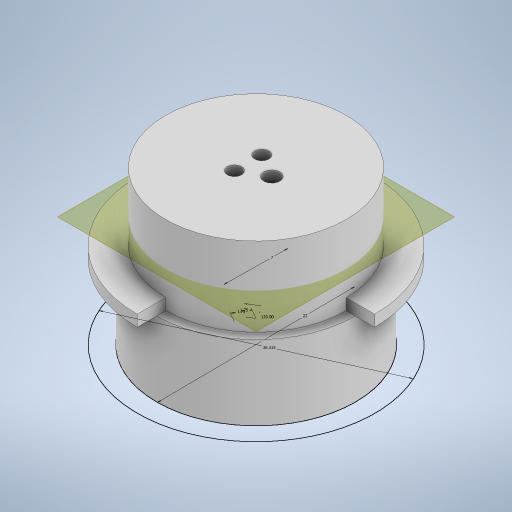
# Autodesk Inventor part: cap
Saved by Autodesk Inventor 2023 (Build 270158000, 158)
## iProperties
Created: 2025-10-02
Part Number: cap
Material: Generic
Document SubType Name: Modeling
Designer: ptato_qo49uko
Density: 1 g/cm^3
Appearance: Default
Author: ptato_qo49uko
Autodesk Inventor part; units mm, degrees
ref_plane "YZ Plane" through (0, 0, 0) normal (1, 0, 0) x (0, 1, 0)
ref_plane "XZ Plane" through (0, 0, 0) normal (0, 1, 0) x (-1, 0, 0)
ref_plane "XY Plane" through (0, 0, 0) normal (0, 0, 1) x (1, 0, 0)
sketch "Sketch1" plane through (0, 0, 0) normal (0, 1, 0) x (-1, 0, 0)
  circle A0 centre (0, 0) radius 11
  circle A1 centre (0, 0) radius 13.1577
  dimension "d0" = 22
  dimension "d40" = 26.3154
  constraints: 2 centre point, 2 coincident
  measures "d0" diameter of A0
  measures "d40" diameter of A1
extrude "Extrusion1" add sketch "Sketch1" along normal blind 17 contours A0
hole "Hole1" at (0, 0, 0) direction (0, 1, 0) diameter 21 depth 7.5
ref_plane "Work Plane1" through (0, 12.25, 0) normal (0, -1, 0) x (1, 0, 0)
sketch "Sketch2" plane through (0, 7.5, 0) normal (0, -1, 0) x (1, 0, 0)
  circle A0 centre (0, 0) radius 3.5
  line L0 (0, 0) -> (2, 0) construction
  line L1 (0, 0) -> (2, 0) construction
  dimension "d10" = 7
  constraints: 4 end point, 2 horizontal, 1 centre point
  measures "d10" diameter of A0
extrude "Extrusion2" add sketch "Sketch2" along normal blind 5
sketch "Sketch3" plane through (0, 2.5, 0) normal (0, -1, 0) x (1, 0, 0)
  line L0 (0, 0) -> (-0.875, -1.5155)
  line L1 (0, 0) -> (1.75, 0) construction
  line L2 (0, 0) -> (-0.875, 1.5155)
  dimension "d19" = 1.75
  dimension "d20" = 120
  dimension "d21" = 1.75
  constraints: 6 end point, 1 equal length, 1 horizontal, 2 other
  measures "d19" distance of L0.start L0.end
  measures "d20" angle of L0 L1
  measures "d21" distance of L0.start L2.end
hole "Hole2" at (-0.875, 2.5, -1.5155) at (-0.875, 2.5, 1.5155) direction (0, 1, 0) diameter 1.6 depth 24
hole "Hole3" at (1.75, 2.5, 0) direction (0, 1, 0) diameter 1.8 depth 23.25
ref_plane "Work Plane2" through (0, 12.25, 0) normal (0, 1, 0) x (1, 0, 0)
extrude "Extrusion3" add sketch "Sketch1" along normal blind 17
extrude "Extrusion4" cut sketch "Sketch1" along normal blind 8.25
sketch "Sketch4" plane through (0, 17, 0) normal (0, 1, 0) x (1, 0, 0)
  circle A0 centre (0, 0) radius 13.1577
  circle A1 centre (0, 0) radius 10
  constraints: 2 centre point, 2 coincident
extrude "Extrusion5" cut sketch "Sketch4" against normal blind 7.5
sketch "Sketch5" plane through (0, 9.5, 0) normal (0, 1, 0) x (1, 0, 0)
  circle A0 centre (0, 0) radius 13.1577 projected
  arc A1 (0, -13.1577) -> (13.1577, 0) centre (0, 0) ccw
  line L0 (13.1577, 0) -> (10, 0)
  circle A2 centre (0, 0) radius 10 projected
  arc A3 (0, 13.1577) -> (-13.1577, 0) centre (0, 0) ccw
  line L1 (-13.1577, 0) -> (-10, 0)
  line L2 (0, 13.1577) -> (0, 10)
  arc A4 (0, -10) -> (10, 0) centre (0, 0) ccw
  arc A5 (0, 10) -> (-10, 0) centre (0, 0) ccw
  line L3 (0, -13.1577) -> (0, -10)
  constraints: 16 point on circle, 8 end point, 5 concentric, 4 centre point, 2 horizontal, 1 perpendicular, 1 vertical
extrude "Extrusion6" cut sketch "Sketch5" against normal blind 1.25 contours A0 L3 A2 L0 | L2 A2 L1 A0
hole "Hole4" at (1.75, 2.5, 0) direction (0, 1, 0) diameter 2.2 depth 2.3
hole "Hole5" at (-0.875, 2.5, 1.5155) at (-0.875, 2.5, -1.5155) direction (0, 1, 0) diameter 1.9 depth 2.3
body "Solid1"
